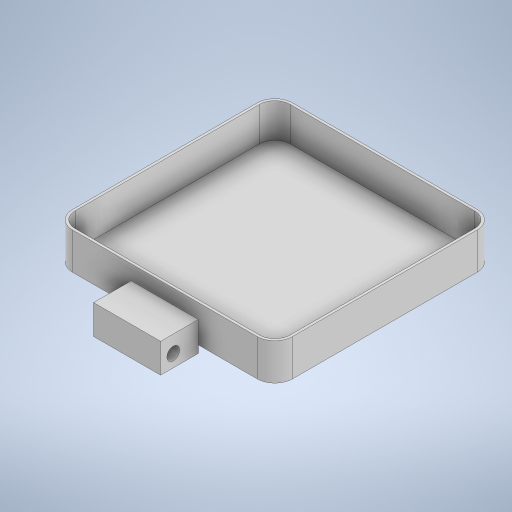
# Autodesk Inventor part: lampa
Saved by Autodesk Inventor 2024 (Build 280153000, 153)
## iProperties
Created: 2023-12-14
Part Number: lampa
Material: Ogólny
Document SubType Name: Modeling
Designer: pient
Density: 1 g/cm^3
Appearance: Domyślna
Author: pient
Autodesk Inventor part; units mm, degrees
ref_plane "YZ Plane" through (0, 0, 0) normal (1, 0, 0) x (0, 1, 0)
ref_plane "XZ Plane" through (0, 0, 0) normal (0, 1, 0) x (-1, 0, 0)
ref_plane "XY Plane" through (0, 0, 0) normal (0, 0, 1) x (1, 0, 0)
sketch "Szkic1" plane through (0, 0, 0) normal (0, 1, 0) x (-1, 0, 0)
  line L0 (52.5, 52.5) -> (-52.5, 52.5)
  line L1 (-52.5, 52.5) -> (-52.5, -52.5)
  line L2 (-52.5, -52.5) -> (52.5, -52.5)
  line L3 (52.5, -52.5) -> (52.5, 52.5)
  point P0 (0, 0)
  dimension "d0" = 105
  dimension "d1" = 105
  dimension "d2" = 52.5
  dimension "d3" = 52.5
  constraints: 8 end point, 2 parallel, 1 horizontal, 1 perpendicular
  measures "d0" distance of L2.end L1.end
  measures "d1" distance of L0.end L1.end
  measures "d2" horizontal distance of L1.end point (0, 0)
  measures "d3" horizontal distance of L1.end point (0, 0)
extrude "Wyciągnięcie proste1" add sketch "Szkic1" along normal blind 17.5
fillet "Zaokrąglenie1" radius 8.5 4 edges at (52.5, 8.75, 52.5) (-52.5, 8.75, 52.5) (52.5, 8.75, -52.5) (-52.5, 8.75, -52.5)
shell "Skorupa1" thickness 1.2 removed faces 1 at (-20.3333, 17.5, -17.5)
sketch "Szkic4" plane through (-44, 0, 52.5) normal (0, 0, 1) x (1, 0, 0)
  line L0 (0, 0) -> (88, 0) projected
  line L1 (28, -3.5) -> (60, -3.5)
  line L2 (60, -3.5) -> (60, 10.5)
  line L3 (60, 10.5) -> (28, 10.5)
  line L4 (28, 10.5) -> (28, -3.5)
  line L5 (0, 17.5) -> (88, 17.5) projected
  point P0 (60, 0)
  point P1 (44, 0)
  point P2 (44, 17.5)
  dimension "d21" = 32
  dimension "d22" = 16
  dimension "d23" = 21
  dimension "d24" = 14
  constraints: 8 end point, 2 midpoint, 2 parallel, 1 horizontal, 1 perpendicular, 1 point on line
  measures "d21" distance of L1.start L1.end
  measures "d22" horizontal distance of L1.end point (44, 0)
  measures "d23" vertical distance of L1.end point (44, 17.5)
  measures "d24" distance of L1.end L2.end
extrude "Wyciągnięcie proste4" add sketch "Szkic4" along normal blind 18
sketch "Szkic6" plane through (-16, -3.5, 52.5) normal (-1, 0, 0) x (0, 0, 1)
  circle A0 centre (12, 6) radius 3
  line L0 (0, 3.5) -> (0, 21) projected
  line L1 (0, 0) -> (18, 0) projected
  point P0 (-52.5, 3.5)
  dimension "d29" = 6
  dimension "d30" = 12
  dimension "d31" = 3
  constraints: 1 centre point
  measures "d29" diameter of A0
  measures "d30" distance from line of L0 A0.centre
  measures "d31" distance edge to line of A0 L1
extrude "Wyciągnięcie proste6" cut sketch "Szkic6" against normal blind 50
